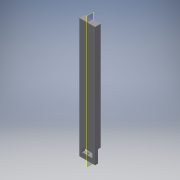
# Autodesk Inventor part: switcher
Saved by Autodesk Inventor 2018 (Build 220112000, 112)
## iProperties
Created: 2017-12-09
Part Number: switcher
Material: Generic
Document SubType Name: Modeling
Designer: ragna
Density: 1 g/cm^3
Appearance: Default
phheight: 5,950 mm
phwidth: 2,500 mm
pheight: 9,100 mm
psnap: 1,700 mm
Author: ragna
Autodesk Inventor part; units mm, degrees
ref_plane "YZ Plane" through (0, 0, 0) normal (1, 0, 0) x (0, 1, 0)
ref_plane "XZ Plane" through (0, 0, 0) normal (0, 1, 0) x (-1, 0, 0)
ref_plane "XY Plane" through (0, 0, 0) normal (0, 0, 1) x (1, 0, 0)
sketch "Sketch8" plane through (0, 0, 0) normal (0, 1, 0) x (-1, 0, 0)
  line L0 (4.55, 0) -> (-4.55, 0)
  line L1 (-4.55, 0) -> (-4.55, -62.26)
  line L2 (-4.55, -62.26) -> (4.55, -62.26)
  line L3 (4.55, -62.26) -> (4.55, 0)
  point P0 (0, 0)
  point P1 (0, 0)
  dimension "d46" = 62.26
  dimension "pheight" = 9.1
  constraints: 8 end point, 2 parallel, 1 coincident, 1 horizontal, 1 midpoint, 1 perpendicular
  measures "d46" distance of L2.end L0.start
  measures "pheight" distance of L0.start L0.end
extrude "Extrusion8" add sketch "Sketch8" along normal blind 3.2
sketch "Sketch9" plane through (4.55, 0, -62.26) normal (0, 0, -1) x (-1, 0, 0)
  line L0 (9.1, 0) -> (9.1, 3.2) projected
  line L1 (0, 0) -> (0, 3.2) projected
  line L2 (9.1, 1.7) -> (0, 1.7)
  line L3 (0, 1.7) -> (0, 0)
  line L4 (0, 0) -> (9.1, 0)
  line L5 (9.1, 0) -> (9.1, 1.7)
  line L6 (0, 3.2) -> (9.1, 3.2) projected
  line L7 (0, 0) -> (9.1, 0) projected
  point P0 (4.55, 0)
  dimension "psnap" = 1.7
  dimension "d65" = 0
  constraints: 8 end point, 2 parallel, 2 point on line, 1 horizontal, 1 perpendicular
  measures "psnap" distance between parallel lines of L2 L4
  measures "d65" distance between parallel lines of L7 L4
extrude "Extrusion9" add sketch "Sketch9" along normal blind 7.24 contours L4 L1 L2 L0
sketch "Sketch10" plane through (-4.55, 0, -62.26) normal (0, 1, 0) x (1, 0, 0)
  line L0 (1.575, 1.93) -> (7.525, 1.93)
  line L1 (7.525, 1.93) -> (7.525, 4.43)
  line L2 (7.525, 4.43) -> (1.575, 4.43)
  line L3 (1.575, 4.43) -> (1.575, 1.93)
  line L4 (0, 7.24) -> (9.1, 7.24) projected
  line L5 (0, -62.26) -> (0, 7.24) projected
  line L6 (9.1, -62.26) -> (9.1, 7.24) projected
  point P0 (4.55, -62.26)
  dimension "phheight" = 5.95
  dimension "phwidth" = 2.5
  dimension "d66" = 2.81
  dimension "d67" = 1.575
  dimension "d68" = 1.575
  constraints: 8 end point, 2 parallel, 1 horizontal, 1 perpendicular
  measures "phheight" distance between parallel lines of L1 L3
  measures "phwidth" distance of L2.end L0.start
  measures "d66" distance between parallel lines of L4 L2
  measures "d67" distance between parallel lines of L5 L3
  measures "d68" distance between parallel lines of L6 L1
extrude "Extrusion10" cut sketch "Sketch10" along normal blind 7
ref_plane "Work Plane2" through (0, 0, 0) normal (-1, 0, 0) x (0, 0, 1)
equation "\"d68\" = d67"
body "Solid2"
